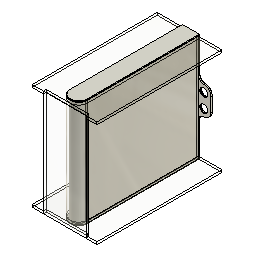
3ChamberBoxOpenTube (Autodesk Fusion 360 design; units mm, degrees)
Autodesk Fusion 360 part; units mm, degrees
sketch "Door" plane through (0, 0, 0) normal (0, 0, 1) x (1, 0, 0)
  line L0 (0, 0) -> (116.205, 0)
  line L1 (116.205, 0) -> (116.205, 224.155)
  line L2 (0, 224.155) -> (0, 0)
  line L3 (20.32, 0) -> (20.32, 5.08)
  line L4 (20.32, 5.08) -> (96.52, 5.08)
  line L5 (96.52, 5.08) -> (96.52, 0)
  line L6 (45.4025, 25.4) -> (42.2275, 25.4)
  line L7 (70.8025, 25.4) -> (73.9775, 25.4)
  arc A0 (45.4025, 25.4) -> (70.8025, 25.4) centre (58.1025, 25.4) ccw
  arc A1 (42.2275, 25.4) -> (73.9775, 25.4) centre (58.1025, 25.4) ccw
  line L8 (42.2275, 25.4) -> (42.2275, 224.155)
  line L9 (45.4025, 25.4) -> (45.4025, 224.155)
  line L10 (73.9775, 25.4) -> (73.9775, 224.155)
  line L11 (70.8025, 25.4) -> (70.8025, 224.155)
  line L12 (116.205, 224.155) -> (70.8025, 224.155)
  line L13 (45.4025, 224.155) -> (0, 224.155)
  dimension "d1" = 116.205
  dimension "d2" = 224.155
  dimension "d3" = 31.75
  dimension "d4" = 25.4
  dimension "d5" = 58.1025
  dimension "d14" = 25.4
  constraint horizontal L0
  constraint vertical L1
  constraint horizontal L12
  constraint vertical L2
  constraint coincident L0.start L2.end
  constraint coincident L0 L3.start
  constraint perpendicular L0 L3
  constraint perpendicular L3 L4
  constraint perpendicular L4 L5
  constraint coincident L0 L5.end
  constraint concentric A0 A1
  constraint horizontal L6
  constraint parallel L6 L7
  constraint tangent A1 L8
  constraint perpendicular L6 L8
  constraint tangent A0 L9
  constraint tangent A1 L10
  constraint perpendicular L7 L10
  constraint tangent A0 L11
  constraint coincident L9.end L12
  constraint coincident L8.end L12
  constraint coincident L10.end L12
  constraint collinear L12 L13
  measures "d1" distance of L0.start L0.end
  measures "d2" distance of L0.start L2.start
  measures "d3" diameter of A1
  measures "d4" distance of L0 A0.centre
  measures "d5" distance of L2 A0.centre
  measures "d14" diameter of A0
extrude "Extrude1" add sketch "Door" along normal blind 4.318 contours L0 L1 L2 L3 L4 L5 A1 L8 L10 L12 L13 makes body 1
extrude "Extrude3" add sketch "Door" against normal blind 194.818 separate body contours L0 L3 L4 L5 makes body 2
copy_body "CopyPasteBodies1" bodies 1 makes body 3
move_body "Move1" bodies 3 to x (1, 0, 0) y (0, 1, 0) z (0, 0, 1) at (0, 0, -194.818)
extrude "Extrude4" add sketch "Door" against normal up to surface (194.818 mm away) separate body contours L6 L7 A0 A1 makes body 4
extrude "Extrude5" add 1 faces at (64.7983, 12.2252, 0) along direction (0, 0, 1) up to surface (4.318 mm away) on bodies 4 bodies 4
move_body "Move2" bodies 3 to x (1, 0, 0) y (0, 1, 0) z (0, 0, 1) at (0, 0, 8.636)
extrude "Extrude6" cut 1 faces at (71.12, 1.6933, -194.818) along direction (0, 0, 1) blind 8.636 on bodies 2 bodies 2
extrude "Extrude7" cut 1 faces at (64.7983, 12.2252, -194.818) along direction (0, 0, 1) blind 8.636 on bodies 4 bodies 4
sketch "Base Plate Etch" plane through (0, 5.08, 0) normal (0, 1, 0) x (-1, 0, 0)
  line L0 (-96.52, -186.182) -> (-20.32, -186.182)
  line L1 (-20.32, -186.182) -> (-20.32, 4.318)
  line L2 (-20.32, 4.318) -> (-96.52, 4.318)
  line L3 (-96.52, 4.318) -> (-96.52, -186.182)
  line L4 (-90.17, -90.932) -> (-26.67, -90.932)
  line L5 (-90.17, -167.132) -> (-26.67, -167.132)
  line L6 (-90.17, -141.732) -> (-26.67, -141.732)
  line L7 (-90.17, -116.332) -> (-26.67, -116.332)
  line L8 (-90.17, -65.532) -> (-26.67, -65.532)
  line L9 (-90.17, -40.132) -> (-26.67, -40.132)
  line L10 (-90.17, -14.732) -> (-26.67, -14.732)
  line L11 (-83.82, -179.832) -> (-33.02, -179.832)
  line L12 (-83.82, -154.432) -> (-33.02, -154.432)
  line L13 (-83.82, -129.032) -> (-33.02, -129.032)
  line L14 (-83.82, -103.632) -> (-33.02, -103.632)
  line L15 (-83.82, -78.232) -> (-33.02, -78.232)
  line L16 (-83.82, -52.832) -> (-33.02, -52.832)
  line L17 (-83.82, -27.432) -> (-33.02, -27.432)
  line L18 (-83.82, -2.032) -> (-33.02, -2.032)
  line L19 (-39.37, -173.482) -> (-77.47, -173.482)
  line L20 (-39.37, -160.782) -> (-77.47, -160.782)
  line L21 (-39.37, -148.082) -> (-77.47, -148.082)
  line L22 (-39.37, -135.382) -> (-77.47, -135.382)
  line L23 (-39.37, -122.682) -> (-77.47, -122.682)
  line L24 (-39.37, -109.982) -> (-77.47, -109.982)
  line L25 (-39.37, -97.282) -> (-77.47, -97.282)
  line L26 (-39.37, -84.582) -> (-77.47, -84.582)
  line L27 (-39.37, -71.882) -> (-77.47, -71.882)
  line L28 (-39.37, -59.182) -> (-77.47, -59.182)
  line L29 (-39.37, -46.482) -> (-77.47, -46.482)
  line L30 (-39.37, -33.782) -> (-77.47, -33.782)
  line L31 (-39.37, -21.082) -> (-77.47, -21.082)
  line L32 (-39.37, -8.382) -> (-77.47, -8.382)
  dimension "d58" = 95.25
  dimension "d59" = 6.35
  dimension "d60" = 6.35
  dimension "d63" = 0
  dimension "d64" = 25.4
  dimension "d65" = 12.7
  dimension "d66" = 12.7
  dimension "d67" = 12.7
  dimension "d70" = 0
  dimension "d71" = 25.4
  dimension "d72" = 6.35
  dimension "d73" = 19.05
  dimension "d74" = 19.05
  dimension "d77" = 0
  dimension "d78" = 12.7
  constraint horizontal L4
  constraint parallel L5 L11
  constraint parallel L11 L19
  measures "d58" distance of L0 L4
  measures "d59" distance of L3 L4.start
  measures "d60" distance of L1 L4.end
  measures "d65" distance of L5 L11
  measures "d66" distance of L3 L11.start
  measures "d67" distance of L1 L11.end
  measures "d72" distance of L5 L19
  measures "d73" distance of L3 L19.end
  measures "d74" distance of L1 L19.start
extrude "Extrude8" add 2 faces at (44.3442, 25.4, -59.182) (71.8608, 25.4, -59.182) along direction (0, 1, 0) up to surface separate body end surface through (42.2275, 224.155, 0) normal (0, 1, 0) offset 0 on bodies 4 makes body 5 at (45.4025, 91.6517, -59.182) makes body 6 at (70.8025, 91.6517, -59.182)
extrude "Extrude9" add 1 faces at (71.12, 1.6933, 0) along direction (0, 0, 1) up to surface (4.318 mm away) separate body on bodies 2 makes body 7
sketch "Tube Side" plane through (0, 0, 0) normal (0, 0, 1) x (1, 0, 0)
  line L0 (45.4025, 224.155) -> (42.2275, 224.155)
  line L1 (42.2275, 227.457) -> (42.2275, 25.4)
  line L2 (42.2275, 25.4) -> (45.4025, 25.4)
  line L3 (45.4025, 25.4) -> (45.4025, 224.155)
  line L4 (73.9775, 224.155) -> (70.8025, 224.155)
  line L5 (70.8025, 224.155) -> (70.8025, 25.4)
  line L6 (70.8025, 25.4) -> (73.9775, 25.4)
  line L7 (73.9775, 25.4) -> (73.9775, 227.457)
  arc A0 (45.4025, 25.4) -> (70.8025, 25.4) centre (58.1025, 25.4) ccw
  line L8 (45.4025, 25.4) -> (42.2275, 25.4)
  arc A1 (42.2275, 25.4) -> (73.9775, 25.4) centre (58.1025, 25.4) ccw
  line L9 (73.9775, 25.4) -> (70.8025, 25.4)
  line L10 (45.4025, 224.155) -> (70.8025, 224.155)
  line L11 (45.5295, 25.4) -> (45.5295, 227.457)
  line L12 (70.6755, 25.4) -> (70.6755, 227.457)
  line L13 (42.2275, 224.282) -> (73.9775, 224.282)
  line L14 (73.9775, 227.457) -> (42.2275, 227.457)
  arc A2 (45.5295, 25.4) -> (70.6755, 25.4) centre (58.1025, 25.4) ccw
  dimension "d83" = 25.146
  dimension "d84" = 0.127
  dimension "d85" = 3.175
  constraint coincident L0.start L3.end
  constraint coincident L4.end L5.start
  constraint concentric A0 A2
  constraint tangent L11 A2
  constraint perpendicular L10 L11
  constraint tangent L12 A2
  constraint perpendicular L10 L12
  constraint parallel L10 L13
  constraint horizontal L14
  constraint coincident L14 L12.end
  constraint coincident L14 L11.end
  constraint coincident L0.end L1
  constraint coincident L1 L13.start
  constraint coincident L4.start L7
  constraint coincident L7 L13.end
  measures "d83" diameter of A2
  measures "d84" distance of L10 L13
  measures "d85" distance of L13 L14
extrude "Extrude13" add sketch "Tube Side" along normal blind 1.6002 separate body makes body 8
move_body "Move5" bodies 8 to x (1, 0, 0) y (0, 1, 0) z (0, 0, 1) at (0, 0, 4.318)
copy_body "CopyPasteBodies3" bodies 8 makes body 9
move_body "Move6" bodies 9 to x (1, 0, 0) y (0, 1, 0) z (0, 0, 1) at (0, 0, -205.74)
move_body "Move7" bodies 9 to x (1, 0, 0) y (0, 1, 0) z (0, 0, 1) at (0, 0, 13.6398)
extrude "Extrude14" add sketch "Tube Side" along normal up to surface (4.318 mm away) contours L10 L11 L12 L13 | L10 L11 L12 A2 | L1 L11 L13 L14 | L11 L12 L13 L14 | L7 L12 L13 L14 bodies 8
extrude "Extrude15" add 1 faces at (62.2935, 91.694, 0) along direction (0, 0, -1) up to surface (186.182 mm away) on bodies 8 bodies 8 9
extrude "Extrude16" add 1 faces at (43.3282, 157.988, -186.182) along direction (0, 0, 1) blind 4.8768 on bodies 8 bodies 8
extrude "Extrude18" cut 1 faces at (43.3282, 157.988, -181.3052) along direction (0, 0, -1) blind 4.8768 on bodies 8 bodies 8
chamfer "Chamfer1" distance 0.8128 angle 45 6 edges at (42.2275, 126.4285, 5.9182) (58.1025, 9.525, 5.9182) (73.9775, 126.4285, 5.9182) (42.2275, 126.4285, -187.7822) (58.1025, 9.525, -187.7822) (73.9775, 126.4285, -187.7822) on bodies 8
sketch "Block-Off" plane through (0, 227.457, 0) normal (0, 1, 0) x (-1, 0, 0)
  line L0 (-73.9775, -186.9694) -> (-73.1647, -187.7822)
  line L1 (-73.1647, -187.7822) -> (-43.0403, -187.7822)
  line L2 (-43.0403, -187.7822) -> (-42.2275, -186.9694)
  line L3 (-42.2275, -186.9694) -> (-42.2275, 5.1054)
  line L4 (-42.2275, 5.1054) -> (-43.0403, 5.9182)
  line L5 (-43.0403, 5.9182) -> (-73.1647, 5.9182)
  line L6 (-73.1647, 5.9182) -> (-73.9775, 5.1054)
  line L7 (-73.9775, 5.1054) -> (-73.9775, -186.9694)
  line L8 (-20.0025, -78.232) -> (-20.0025, -103.632)
  line L9 (-96.2025, -103.632) -> (-96.2025, -78.232)
  line L10 (-96.2025, -65.532) -> (-20.0025, -116.332) construction
  line L11 (-20.0025, -65.532) -> (-96.2025, -116.332) construction
  arc A0 (-96.2025, -103.632) -> (-83.5025, -116.332) centre (-83.5025, -103.632) ccw
  arc A1 (-83.5025, -65.532) -> (-96.2025, -78.232) centre (-83.5025, -78.232) ccw
  arc A2 (-20.0025, -78.232) -> (-32.7025, -65.532) centre (-32.7025, -78.232) ccw
  arc A3 (-32.7025, -116.332) -> (-20.0025, -103.632) centre (-32.7025, -103.632) ccw
  circle A4 centre (-83.5025, -103.632) radius 6.35
  circle A5 centre (-83.5025, -78.232) radius 6.35
  circle A6 centre (-32.7025, -103.632) radius 6.35
  circle A7 centre (-32.7025, -78.232) radius 6.35
  line L12 (-32.7025, -116.332) -> (-42.2275, -116.332)
  line L13 (-73.9775, -116.332) -> (-83.5025, -116.332)
  line L14 (-83.5025, -65.532) -> (-73.9775, -65.532)
  line L15 (-42.2275, -65.532) -> (-32.7025, -65.532)
  point P0 (-58.1025, -90.932)
  dimension "d108" = 76.2
  dimension "d109" = 50.8
  dimension "d110" = 12.7
  dimension "d111" = 12.7
  dimension "d112" = 12.7
  dimension "d113" = 12.7
  dimension "d114" = 12.7
  constraint horizontal L14
  constraint perpendicular L8 L14
  constraint parallel L12 L14
  constraint parallel L8 L9
  constraint coincident L10 P0
  constraint coincident L11 P0
  constraint coincident L11.end L9
  constraint coincident L11.end L12
  constraint tangent L9 A0
  constraint tangent A0 L12
  constraint coincident L10.start L14
  constraint coincident L10.start L9
  constraint tangent A1 L14
  constraint tangent L9 A1
  constraint equal A0 A1
  constraint coincident L11.start L14
  constraint coincident L11.start L8
  constraint tangent A2 L14
  constraint tangent L8 A2
  constraint equal A0 A2
  constraint coincident L10.end L8
  constraint coincident L10.end L12
  constraint tangent L8 A3
  constraint tangent A3 L12
  constraint equal A0 A3
  constraint concentric A0 A4
  constraint concentric A1 A5
  constraint concentric A3 A6
  constraint concentric A2 A7
  constraint coincident L3 L12.end
  constraint coincident L7 L13.start
  constraint collinear L12 L13
  constraint coincident L7 L14.end
  constraint coincident L3 L15.start
  constraint collinear L14 L15
  measures "d108" distance of L10.end L11.end
  measures "d109" distance of L11.start L10.end
  measures "d110" radius of A0
  measures "d111" diameter of A4
  measures "d112" diameter of A5
  measures "d113" diameter of A6
  measures "d114" diameter of A7
extrude "Extrude19" add sketch "Block-Off" against normal up to surface (3.175 mm away) contours L7 L9 A0 A1 L13 L14 | L3 L8 A2 A3 L12 L15 bodies 8
fillet "Fillet1" radius 9.525 4 edges at (42.2275, 225.8695, -65.532) (42.2275, 225.8695, -116.332) (73.9775, 225.8695, -116.332) (73.9775, 225.8695, -65.532) on bodies 8
chamfer "Chamfer2" distance 0.8128 angle 45 20 edges at (58.1025, 227.457, -187.7822) (42.6339, 227.457, -187.3758) (73.5711, 227.457, -187.3758) (73.9775, 227.457, -156.4132) (76.7673, 227.457, -119.1218) (92.4828, 227.457, -112.6123) (96.2025, 227.457, -90.932) (92.4828, 227.457, -69.2517) (76.7673, 227.457, -62.7422) (73.9775, 227.457, -25.4508) (42.2275, 227.457, -156.4132) (39.4377, 227.457, -119.1218) (23.7222, 227.457, -112.6123) (20.0025, 227.457, -90.932) (23.7222, 227.457, -69.2517) (39.4377, 227.457, -62.7422) (42.2275, 227.457, -25.4508) (42.6339, 227.457, 5.5118) (58.1025, 227.457, 5.9182) (73.5711, 227.457, 5.5118) on bodies 8
chamfer "Chamfer3" distance 0.8128 angle 45 8 edges at (89.4228, 227.457, -101.3357) (89.4228, 224.282, -101.3357) (89.4228, 227.457, -75.9357) (89.4228, 224.282, -75.9357) (38.6228, 227.457, -75.9357) (38.6228, 224.282, -75.9357) (38.6228, 227.457, -101.3357) (38.6228, 224.282, -101.3357) on bodies 8
combine "Combine5" operation add target body 2 tool bodies 7
sketch "Doors Cut" plane through (0, 0, 4.318) normal (0, 0, 1) x (-1, 0, 0)
  arc A0 (-42.2275, -25.4) -> (-73.9775, -25.4) centre (-58.1025, -25.4) ccw
  line L0 (-42.2275, -25.4) -> (-42.2275, -224.155)
  line L1 (-42.2275, -224.155) -> (0, -224.155)
  line L2 (0, -224.155) -> (0, 0)
  line L3 (0, 0) -> (-20.32, 0)
  line L4 (-20.32, 0) -> (-20.32, -5.08)
  line L5 (-20.32, -5.08) -> (-96.52, -5.08)
  line L6 (-96.52, -5.08) -> (-96.52, 0)
  line L7 (-96.52, 0) -> (-116.205, 0)
  line L8 (-116.205, 0) -> (-116.205, -224.155)
  line L9 (-116.205, -224.155) -> (-73.9775, -224.155)
  line L10 (-73.9775, -224.155) -> (-73.9775, -25.4)
sketch "Base Cut" plane through (0, 5.08, 0) normal (0, 1, 0) x (-1, 0, 0)
  line L0 (-96.52, -186.182) -> (-20.32, -186.182)
  line L1 (-20.32, -186.182) -> (-20.32, 4.318)
  line L2 (-20.32, 4.318) -> (-96.52, 4.318)
  line L3 (-96.52, 4.318) -> (-96.52, -186.182)
sketch "Tube Walls Cut" plane through (42.2275, 0, 0) normal (-1, 0, 0) x (0, -1, 0)
  line L0 (-224.155, 4.318) -> (-224.155, -186.182)
  line L1 (-224.155, -186.182) -> (-25.4, -186.182)
  line L2 (-25.4, -186.182) -> (-25.4, 4.318)
  line L3 (-25.4, 4.318) -> (-224.155, 4.318)
equation "d5 = ( 4.575 / 2 ) * 1 in"
equation "d12 = -7.5 in - 0.170 in"
equation "d58 = ( 7.5 / 2 ) * 1 in"
equation "d101 = 0.255 in - 0.063 in"
named bodies: "Door 1", "Door 2", "Tube Bottom", "Left Tube Wall", "Right Tube Wall", "Block-Off", "Base Plate"
